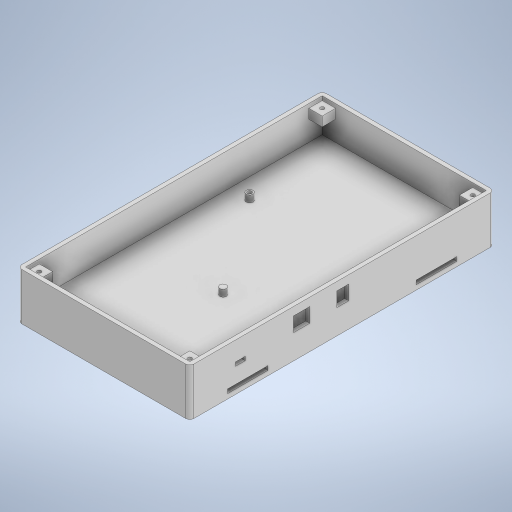
# Autodesk Inventor part: Base
Saved by Autodesk Inventor 2023 (Build 270158000, 158)
## iProperties
Created: 2023-01-13
Part Number: Base
Material: Generic
Document SubType Name: Modeling
Designer: Ahmed Nazir
Density: 1 g/cm^3
Appearance: Default
Author: Ahmed Nazir
Autodesk Inventor part; units mm, degrees
ref_plane "YZ Plane" through (0, 0, 0) normal (1, 0, 0) x (0, 1, 0)
ref_plane "XZ Plane" through (0, 0, 0) normal (0, 1, 0) x (-1, 0, 0)
ref_plane "XY Plane" through (0, 0, 0) normal (0, 0, 1) x (1, 0, 0)
sketch "Sketch1" plane through (0, 0, 0) normal (0, 1, 0) x (-1, 0, 0)
  line L0 (0, 0) -> (121.76, 0)
  line L1 (121.76, 0) -> (121.76, -220)
  line L2 (121.76, -220) -> (0, -220)
  line L3 (0, -220) -> (0, 0)
  line L4 (124.76, -223) -> (124.76, 3)
  line L5 (124.76, 3) -> (-3, 3)
  line L6 (-3, 3) -> (-3, -223)
  line L7 (-3, -223) -> (124.76, -223)
  circle A0 centre (5.08, -10.08) radius 1.6
  circle A1 centre (5.08, -10.08) radius 2.6
  circle A2 centre (55.88, -80.565) radius 2.5
  circle A3 centre (5.08, -151.05) radius 1.6
  circle A4 centre (5.08, -151.05) radius 2.6
  circle A5 centre (106.68, -10.08) radius 1.6
  circle A6 centre (106.68, -10.08) radius 2.6
  circle A7 centre (106.68, -151.05) radius 1.6
  circle A8 centre (106.68, -151.05) radius 2.6
  dimension "d0" = 121.76
  dimension "d1" = 220
  dimension "d2" = 3
  dimension "d22" = 3.2
  dimension "d23" = 1
  dimension "d24" = 5.08
  dimension "d25" = 10.08
  dimension "d26" = 5
  dimension "d35" = 3.2
  dimension "d36" = 1
  dimension "d37" = 140.97
  dimension "d38" = 0
  dimension "d39" = 3.2
  dimension "d40" = 1
  dimension "d41" = 101.6
  dimension "d42" = 0
  dimension "d43" = 3.2
  dimension "d44" = 1
  dimension "d45" = 0
  dimension "d46" = 0
  dimension "d47" = 50.8
  dimension "d48" = 70.485
  constraints: 16 end point, 9 centre point, 4 parallel, 2 perpendicular, 1 horizontal, 3 other
  measures "d0" distance of L1.end L2.end
  measures "d1" distance of L0.end L1.end
  measures "d2" distance between parallel lines of L1 L4
  measures "d22" diameter of A0
  measures "d23" radial gap between concentric circles of A0 A1
  measures "d24" distance from line of L3 A0.centre
  measures "d25" distance from line of A0.centre L0
  measures "d26" diameter of A2
  measures "d35" diameter of A3
  measures "d36" radial gap between concentric circles of A3 A4
  measures "d37" distance of A3.centre A0.centre
  measures "d38" horizontal distance of A3.centre A0.centre
  measures "d39" diameter of A5
  measures "d40" radial gap between concentric circles of A5 A6
  measures "d41" distance of A0.centre A5.centre
  measures "d42" vertical distance of A5.centre A0.centre
  measures "d43" diameter of A7
  measures "d44" radial gap between concentric circles of A7 A8
  measures "d45" vertical distance of A3.centre A7.centre
  measures "d46" horizontal distance of A5.centre A7.centre
  measures "d47" horizontal distance of A2.centre A0.centre
  measures "d48" vertical distance of A2.centre A5.centre
extrude "Extrusion1" add sketch "Sketch1" along normal blind 10 contours L0 L1 L2 L3 | A0 | A1 | A2 | A3 | A4 | A5 | A6 | A7 | A8
extrude "Extrusion2" add sketch "Sketch1" along normal blind 35 contours L7 L6 L5 L4
fillet "Fillet1" radius 3 4 edges at (3, 17.5, -223) (-124.76, 17.5, -223) (-124.76, 17.5, 3) (3, 17.5, 3)
sketch "Sketch2" plane through (3, 0, 0) normal (1, 0, 0) x (0, 0, -1)
  line L0 (220, 10) -> (0, 10) construction
  line L1 (0, 10) -> (220, 10)
  line L2 (73.9, 28.95) -> (86, 28.95)
  line L3 (86, 28.95) -> (86, 18.2)
  line L4 (86, 18.2) -> (73.9, 18.2)
  line L5 (73.9, 18.2) -> (73.9, 28.95)
  line L6 (106.15, 28.95) -> (114.9, 28.95)
  line L7 (114.9, 28.95) -> (114.9, 18.2)
  line L8 (114.9, 18.2) -> (106.15, 18.2)
  line L9 (106.15, 18.2) -> (106.15, 28.95)
  line L10 (0, 0) -> (0, 35) projected
  line L11 (30.85, 20.9) -> (38.15, 20.9)
  line L12 (38.15, 20.9) -> (38.15, 18.1)
  line L13 (38.15, 18.1) -> (30.85, 18.1)
  line L14 (30.85, 18.1) -> (30.85, 20.9)
  line L15 (25, 6.5) -> (55, 6.5)
  line L16 (55, 6.5) -> (55, 3.5)
  line L17 (55, 3.5) -> (25, 3.5)
  line L18 (25, 3.5) -> (25, 6.5)
  line L19 (110, 10) -> (110, 0) construction
  line L20 (220, 0) -> (0, 0) projected
  line L21 (195, 6.5) -> (165, 6.5)
  line L22 (165, 6.5) -> (165, 3.5)
  line L23 (165, 3.5) -> (195, 3.5)
  line L24 (195, 3.5) -> (195, 6.5)
  dimension "d9" = 12.1
  dimension "d10" = 10.75
  dimension "d11" = 8.2
  dimension "d12" = 8.75
  dimension "d13" = 10.75
  dimension "d14" = 8.2
  dimension "d15" = 20.15
  dimension "d19" = 7.3
  dimension "d20" = 2.8
  dimension "d21" = 8.1
  dimension "d29" = 30
  dimension "d30" = 3
  dimension "d31" = 3.5
  dimension "d32" = 25
  dimension "d49" = 35.75
  dimension "d50" = 30.85
  constraints: 44 end point, 9 equal length, 4 horizontal, 4 perpendicular, 4 symmetric about line, 2 midpoint
  measures "d9" distance of L3.end L4.end
  measures "d10" distance of L2.end L3.end
  measures "d11" distance between parallel lines of L0 L4
  measures "d12" distance of L7.end L8.end
  measures "d13" distance of L6.end L7.end
  measures "d14" distance between parallel lines of L0 L8
  measures "d15" distance between parallel lines of L9 L3
  measures "d19" distance of L12.end L13.end
  measures "d20" distance of L11.end L12.end
  measures "d21" distance between parallel lines of L0 L13
  measures "d29" distance of L16.end L17.end
  measures "d30" distance of L15.end L16.end
  measures "d31" distance between parallel lines of L0 L15
  measures "d32" distance between parallel lines of L10 L18
  measures "d49" distance between parallel lines of L5 L12
  measures "d50" distance between parallel lines of L10 L14
extrude "Extrusion3" cut sketch "Sketch2" against normal up to surface (3 mm away) contours L2 L3 L4 L5 | L6 L7 L8 L9 | L11 L12 L13 L14
extrude "Extrusion4" add sketch "Sketch1" along normal blind 15 contours A1 | A2 | A4 | A6 | A8
extrude "Extrusion5" cut sketch "Sketch2" against normal through all contours L15 L16 L17 L18 | L24 L23 L22 L21
sketch "Sketch3" plane through (0, 35, 0) normal (0, 1, 0) x (1, 0, 0)
  line L0 (-121.76, 0) -> (-121.76, 220) projected
  line L1 (-121.76, 110) -> (0, 110) construction
  line L2 (0, 220) -> (0, 0) projected
  line L3 (-121.76, 0) -> (0, 0) projected
  line L4 (-60.88, 0) -> (-60.88, 220) construction
  line L5 (-121.76, 220) -> (0, 220) projected
  line L6 (0, 0) -> (-10, 0)
  line L7 (-10, 0) -> (-10, 10)
  line L8 (-10, 10) -> (0, 10)
  line L9 (0, 10) -> (0, 0)
  line L10 (-121.76, 0) -> (-111.76, 0)
  line L11 (-111.76, 0) -> (-111.76, 10)
  line L12 (-111.76, 10) -> (-121.76, 10)
  line L13 (-121.76, 10) -> (-121.76, 0)
  line L14 (0, 220) -> (-10, 220)
  line L15 (-10, 220) -> (-10, 210)
  line L16 (-10, 210) -> (0, 210)
  line L17 (0, 210) -> (0, 220)
  line L18 (-121.76, 220) -> (-111.76, 220)
  line L19 (-111.76, 220) -> (-111.76, 210)
  line L20 (-111.76, 210) -> (-121.76, 210)
  line L21 (-121.76, 210) -> (-121.76, 220)
  line L22 (-121.76, 0) -> (0, 0)
  line L23 (0, 0) -> (0, 220)
  line L24 (0, 220) -> (-121.76, 220)
  line L25 (-121.76, 220) -> (-121.76, 0)
  point P0 (0, 210)
  dimension "d51" = 10
  dimension "d52" = 10
  constraints: 44 end point, 9 symmetric about line, 4 midpoint, 4 parallel, 2 horizontal, 2 perpendicular
  measures "d51" distance of L7.end L8.end
  measures "d52" distance of L6.end L7.end
extrude "Extrusion6" add sketch "Sketch3" against normal blind 10 contours L0 L12 L11 L3 | L0 L5 L19 L20 | L7 L8 L2 L3 | L5 L2 L16 L15
sketch "Sketch4" plane through (0, 35, 0) normal (0, 1, 0) x (1, 0, 0)
  line L0 (-10, 10) -> (-10, 0) projected
  line L1 (0, 10) -> (-10, 10) projected
  line L2 (-10, 220) -> (-10, 210) projected
  line L3 (-10, 210) -> (0, 210) projected
  line L4 (-121.76, 210) -> (-111.76, 210) projected
  line L5 (-111.76, 210) -> (-111.76, 220) projected
  line L6 (-111.76, 0) -> (-111.76, 10) projected
  line L7 (-111.76, 10) -> (-121.76, 10) projected
  point P0 (0, 0)
  point P1 (-5, 5)
  point P2 (-116.76, 5)
  point P3 (-116.76, 215)
  point P4 (-5, 215)
  dimension "d55" = 5
  dimension "d63" = 5
  dimension "d64" = 5
  dimension "d65" = 5
  dimension "d66" = 5
  dimension "d67" = 5
  dimension "d68" = 5
  dimension "d69" = 5
  measures "d55" distance from line of L0 point (-5, 5)
  measures "d63" distance from line of L1 point (-5, 5)
  measures "d64" distance from line of L2 point (-5, 215)
  measures "d65" distance from line of L3 point (-5, 215)
  measures "d66" distance from line of L4 point (-116.76, 215)
  measures "d67" distance from line of L5 point (-116.76, 215)
  measures "d68" distance from line of L6 point (-116.76, 5)
  measures "d69" distance from line of L7 point (-116.76, 5)
hole "Hole1" at (-5, 35, -5) at (-5, 35, -215) at (-116.76, 35, -215) at (-116.76, 35, -5) direction (0, -1, 0) diameter 3 depth 10
extrude "Extrusion7" cut sketch "Sketch3" against normal blind 3
body "Solid1"
